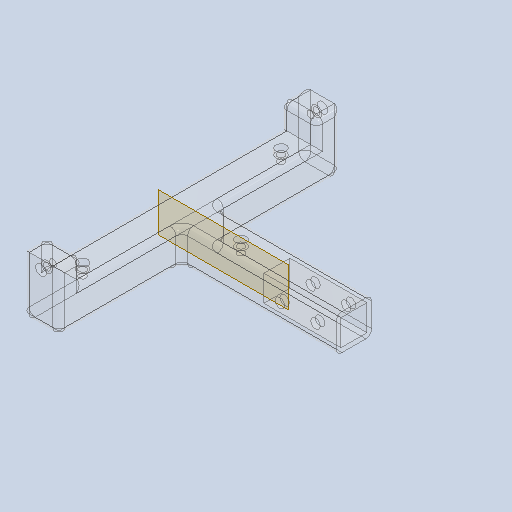
# Autodesk Inventor part: e
Saved by Autodesk Inventor 2025.3 (Build 293356000, 356)
## iProperties
Created: 2026-04-18
Part Number: e
Material: PCTG 20%
Document SubType Name: Modeling
Designer: ksawe
Density: 1.541 g/cm^3
Appearance: Polycarbonate - Clear(1)
Author: ksawe
Autodesk Inventor part; units mm, degrees
ref_plane "YZ Plane" through (0, 0, 0) normal (1, 0, 0) x (0, 1, 0)
ref_plane "XZ Plane" through (0, 0, 0) normal (0, 1, 0) x (-1, 0, 0)
ref_plane "XY Plane" through (0, 0, 0) normal (0, 0, 1) x (1, 0, 0)
sketch "Sketch1" plane through (0, 0, 0) normal (0, 1, 0) x (-1, 0, 0)
  line L0 (15, 118.75) -> (-15, 118.75)
  line L1 (-15, -118.75) -> (15, -118.75)
  line L2 (15, -118.75) -> (15, 118.75)
  line L3 (15, 118.75) -> (-15, -118.75) construction
  line L4 (-15, 118.75) -> (15, -118.75) construction
  line L5 (-15, 15) -> (-145.33, 15)
  line L6 (15, 0) -> (-145.33, 0) construction
  line L7 (-15, -15) -> (-145.33, -15)
  line L8 (-145.33, 15) -> (-145.33, -15)
  line L9 (-15, 118.75) -> (-15, 15)
  line L10 (-15, -15) -> (-15, -118.75)
  point P0 (0, 0)
  dimension "d0" = 30
  dimension "d1" = 237.5
  dimension "d2" = 15
  dimension "d3" = 130.33
  constraints: 22 end point, 4 midpoint, 4 perpendicular, 3 parallel, 2 coincident, 2 horizontal, 2 horizontal alignment, 2 symmetric about line, 1 vertical
  measures "d0" distance of L1.end L1.start
  measures "d1" distance of L1.end L0.start
  measures "d2" distance between parallel lines of L6 L7
  measures "d3" distance of L7.start L7.end
extrude "Extrusion1" add sketch "Sketch1" along normal blind 30
ref_plane "Work Plane1" through (15, 0, 0) normal (0, 0, 1) x (1, 0, 0)
sketch "Sketch2" plane through (0, 30, 0) normal (0, 1, 0) x (1, 0, 0)
  line L0 (-15, 118.75) -> (-15, -118.75) projected
  line L1 (15, -118.75) -> (15, -15) projected
  line L2 (-15, -118.75) -> (15, -118.75)
  line L3 (15, -118.75) -> (15, -98.75)
  line L4 (15, -98.75) -> (-15, -98.75)
  line L5 (-15, -98.75) -> (-15, -118.75)
  point P0 (0, 0)
  point P1 (15, -118.75)
  point P2 (-15, -98.75)
  dimension "d6" = 20
  constraints: 8 end point, 2 parallel, 2 vertical alignment, 1 horizontal, 1 perpendicular, 1 point on line
  measures "d6" distance between parallel lines of L4 L2
extrude "Extrusion2" add sketch "Sketch2" along normal blind 20
sketch "Sketch3" plane through (-15, 0, 118.75) normal (0, 0, 1) x (1, 0, 0)
  line L0 (0, 50) -> (30, 50) projected
  line L1 (30, 0) -> (30, 50) projected
  point P0 (15, 0)
  point P1 (15, 42)
  dimension "d9" = 8
  dimension "d10" = 15
  measures "d9" distance from line of L0 point (15, 42)
  measures "d10" distance from line of L1 point (15, 42)
hole "Hole1" at (0, 42, 118.75) direction (0, 0, -1) diameter 6 depth 10 tip angle 118 counterbore diameter 9 counterbore depth 5
mirror "Mirror1" about plane through (15, 0, 0) normal (0, 0, 1) of "Extrusion2", "Hole1"
sketch "Sketch4" plane through (145.33, 0, 15) normal (1, 0, 0) x (0, 0, -1)
  line L0 (0, 0) -> (30, 0) projected
  line L1 (30, 0) -> (30, 30) projected
  line L2 (0, 30) -> (30, 30) projected
  line L3 (0, 0) -> (0, 30) projected
  line L4 (4, 26) -> (26, 26)
  line L5 (26, 26) -> (26, 4)
  line L6 (26, 4) -> (4, 4)
  line L7 (4, 4) -> (4, 26)
  point P0 (15, 0)
  constraints: 8 end point, 3 other
extrude "Extrusion3" cut sketch "Sketch4" against normal blind 65 contours L4 L5 L6 L7
sketch "Sketch5" plane through (15, 0, 15) normal (0, 0, 1) x (1, 0, 0)
  line L0 (65.33, 4) -> (65.33, 26) projected
  circle A0 centre (82.83, 15) radius 4
  circle A1 centre (112.83, 15) radius 4
  point P0 (-15, 0)
  point P1 (65.33, 15)
  dimension "d20" = 8
  dimension "d21" = 8
  dimension "d22" = 30
  dimension "d23" = 17.5
  constraints: 2 centre point, 2 horizontal alignment, 1 midpoint
  measures "d20" diameter of A0
  measures "d21" diameter of A1
  measures "d22" distance of A1.centre A0.centre
  measures "d23" distance from line of L0 A0.centre
extrude "Extrusion4" cut sketch "Sketch5" against normal through all
fillet "Fillet1" radius 5 28 edges at (15, 15, 15) (15, 15, -15) (80.165, 0, 15) (80.165, 0, -15) (80.165, 30, -15) (80.165, 30, 15) (15, 30, 56.875) (15, 30, -56.875) (15, 0, -66.875) (15, 0, 66.875) (15, 25, 118.75) (-15, 25, 118.75) (0, 0, 118.75) (-15, 0, 0) (0, 0, -118.75) (15, 25, -118.75) (-15, 25, -118.75) (-15, 30, 0) (15, 50, 108.75) (-15, 50, 108.75) (0, 50, 98.75) (-15, 40, 98.75) (15, 40, 98.75) (15, 40, -98.75) (0, 50, -98.75) (15, 50, -108.75) (-15, 50, -108.75) (-15, 40, -98.75)
sketch "Sketch6" plane through (0, 30, 0) normal (0, 1, 0) x (1, 0, 0)
  line L0 (-10, -98.75) -> (-10, 98.75) projected
  line L1 (-10, -98.75) -> (10, -98.75) projected
  point P0 (0, 0)
  point P1 (0, -83.75)
  dimension "d27" = 10
  dimension "d35" = 15
  measures "d27" distance from line of L0 point (0, -83.75)
  measures "d35" distance from line of L1 point (0, -83.75)
hole "Hole2" at (0, 30, 83.75) direction (0, -1, 0) diameter 6 depth 10 tip angle 118 counterbore diameter 9 counterbore depth 5
sketch "Sketch7" plane through (0, 30, 0) normal (0, 1, 0) x (1, 0, 0)
  line L0 (20, 10) -> (145.33, 10) projected
  line L1 (-10, -98.75) -> (-10, 98.75) projected
  line L2 (10, 98.75) -> (-10, 98.75) projected
  point P0 (0, 0)
  point P1 (0, 83.75)
  point P2 (50, 0)
  dimension "d36" = 10
  dimension "d44" = 60
  dimension "d45" = 10
  dimension "d46" = 15
  measures "d36" distance from line of L0 point (50, 0)
  measures "d44" distance from line of L1 point (50, 0)
  measures "d45" distance from line of L1 point (0, 83.75)
  measures "d46" distance from line of L2 point (0, 83.75)
hole "Hole3" at (50, 30, 0) at (0, 30, -83.75) direction (0, -1, 0) diameter 6 depth 10 tip angle 118 counterbore diameter 9 counterbore depth 5
body "Solid1"
